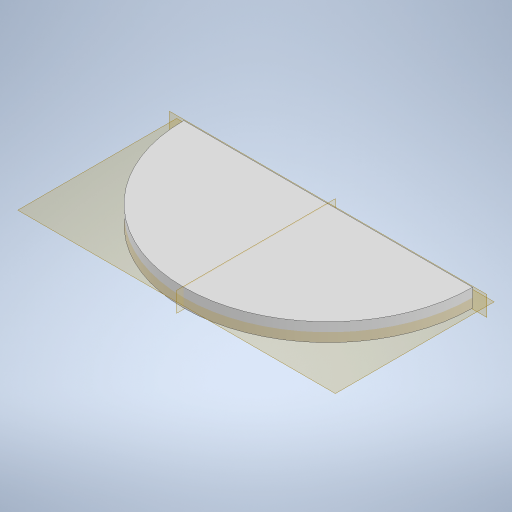
# Autodesk Inventor part: Веер
Saved by Autodesk Inventor 2023.2 (Build 272271030, 271C)
## iProperties
Created: 2024-01-31
Part Number: Веер
Material: Типовые
Document SubType Name: Modeling
Designer: I9232
Density: 1 g/cm^3
Appearance: По умолчанию
Author: I9232
Autodesk Inventor part; units mm, degrees
sketch "Эскиз2" plane through (0, 0, 0) normal (0, 1, 0) x (-1, 0, 0)
  line L0 (200, 0) -> (-200, 0)
  arc A0 (200, 0) -> (-200, 0) centre (0, 0) ccw
  dimension "d0" = 400
  dimension "d1" = 200
  constraints: 2 end point, 2 point on circle, 1 centre point, 1 coincident, 1 horizontal
  measures "d0" distance of L0.start L0.end
  measures "d1" radius of A0
extrude "Выдавливание1" add sketch "Эскиз2" along normal mid plane 25
